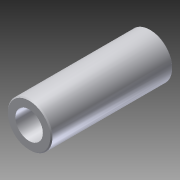
# Autodesk Inventor part: am-0243
Saved by Autodesk Inventor 2012 (Build 160160000, 160)
## iProperties
Category: Chassis
Company: Autodesk Inc.
Created: 2011-12-22
Part Number: am-0243
Document SubType Name: Modeling
Designer: Autodesk Inc.
Density: 1 g/cm^3
Catalog Web Link: http://www.andymark.com/product-p/am-0243.htm
Vendor: Andy Mark Inc.
Material: Default
Author: Autodesk Inc.
Autodesk Inventor part; units mm, degrees
ref_plane "YZ Plane" through (0, 0, 0) normal (1, 0, 0) x (0, 1, 0)
ref_plane "XZ Plane" through (0, 0, 0) normal (0, 1, 0) x (-1, 0, 0)
ref_plane "XY Plane" through (0, 0, 0) normal (0, 0, 1) x (1, 0, 0)
sketch "Sketch1" plane through (0, 0, 0) normal (0, 0, 1) x (1, 0, 0)
  circle A0 centre (0, 0) radius 5.334
  circle A1 centre (0, 0) radius 8.636
  dimension "d0" = 10.668
  dimension "d1" = 17.272
  constraints: 2 centre point, 2 coincident
  measures "d0" diameter of A0
  measures "d1" diameter of A1
extrude "Extrusion1" add sketch "Sketch1" against normal blind 47.244
chamfer "Chamfer1" distance 0.3969 angle 45 2 edges at (-8.636, 0, 0) (-8.636, 0, -47.244)
body "Solid1"
